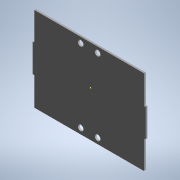
# Autodesk Inventor part: Level1
Saved by Autodesk Inventor 2020 (Build 240168000, 168)
## iProperties
Part Number: Level1
Material: Generic
Document SubType Name: Modeling
Designer: SBBA
Appearance: Default
Mass: 86.85 g
Surface Area: 601.8 cm^2
Volume: 86.85 cm^3
Density: 1 g/cm^3
Author: SBBA
Autodesk Inventor part; units mm, degrees
ref_plane "YZ Plane" through (0, 0, 0) normal (1, 0, 0) x (0, 1, 0)
ref_plane "XZ Plane" through (0, 0, 0) normal (0, 1, 0) x (-1, 0, 0)
ref_plane "XY Plane" through (0, 0, 0) normal (0, 0, 1) x (1, 0, 0)
sketch "Sketch1" plane through (0, 0, 0) normal (0, 0, 1) x (1, 0, 0)
  line L0 (-102.5157, 69.2842) -> (97.4843, 69.2842)
  line L1 (97.4843, 69.2842) -> (97.4843, -80.7158)
  line L2 (97.4843, -80.7158) -> (-102.5157, -80.7158)
  line L3 (-102.5157, -80.7158) -> (-102.5157, 69.2842)
  point P0 (0, 0)
  constraints: 8 end point, 2 parallel, 1 horizontal, 1 perpendicular
extrude "Extrusion1" add sketch "Sketch1" along normal blind 3
sketch "Sketch3" plane through (0, 0, 3) normal (0, 0, 1) x (1, 0, 0)
  point P0 (0, 0)
sketch "Sketch4" plane through (0, 0, 3) normal (0, 0, 1) x (1, 0, 0)
  line L0 (97.4843, 69.2842) -> (-102.5157, 69.2842) projected
  line L1 (-102.5157, 69.2842) -> (-99.5157, 69.2842)
  line L2 (-99.5157, 69.2842) -> (-99.5157, 19.2842)
  line L3 (-99.5157, 19.2842) -> (-102.5157, 19.2842)
  line L4 (-102.5157, 19.2842) -> (-102.5157, 69.2842)
  point P0 (0, 0)
  constraints: 8 end point, 2 parallel, 1 horizontal, 1 perpendicular
extrude "Extrusion2" cut sketch "Sketch4" against normal blind 3
sketch "Sketch5" plane through (0, 0, 3) normal (0, 0, 1) x (1, 0, 0)
  line L0 (97.4843, -80.7158) -> (94.4843, -80.7158)
  line L1 (94.4843, -80.7158) -> (94.4843, -30.7158)
  line L2 (94.4843, -30.7158) -> (97.4843, -30.7158)
  line L3 (97.4843, -30.7158) -> (97.4843, -80.7158)
  point P0 (0, 0)
  point P1 (-102.5157, -80.7158)
  dimension "d17" = 3
  dimension "d18" = 50
  constraints: 8 end point, 2 parallel, 1 horizontal, 1 perpendicular
  measures "d17" distance of L1.end L2.end
  measures "d18" distance of L2.end L0.start
extrude "Extrusion3" cut sketch "Sketch5" against normal blind 3
sketch "Sketch6" plane through (0, 0, 3) normal (0, 0, 1) x (1, 0, 0)
  line L0 (97.4843, -30.7158) -> (97.4843, 69.2842) projected
  line L1 (97.4843, 69.2842) -> (94.4843, 69.2842)
  line L2 (94.4843, 69.2842) -> (94.4843, 19.2842)
  line L3 (94.4843, 19.2842) -> (97.4843, 19.2842)
  line L4 (97.4843, 19.2842) -> (97.4843, 69.2842)
  point P0 (0, 0)
  dimension "d21" = 50
  dimension "d22" = 3
  constraints: 8 end point, 2 parallel, 1 horizontal, 1 perpendicular
  measures "d21" distance of L1.end L2.end
  measures "d22" distance of L0.end L1.end
extrude "Extrusion4" cut sketch "Sketch6" against normal blind 3
sketch "Sketch7" plane through (0, 0, 3) normal (0, 0, 1) x (1, 0, 0)
  line L0 (-102.5157, 19.2842) -> (-102.5157, -80.7158) projected
  line L1 (-102.5157, -80.7158) -> (-99.5157, -80.7158)
  line L2 (-99.5157, -80.7158) -> (-99.5157, -30.7158)
  line L3 (-99.5157, -30.7158) -> (-102.5157, -30.7158)
  line L4 (-102.5157, -30.7158) -> (-102.5157, -80.7158)
  point P0 (0, 0)
  dimension "d25" = 50
  dimension "d26" = 3
  constraints: 8 end point, 2 parallel, 1 horizontal, 1 perpendicular
  measures "d25" distance of L1.end L2.end
  measures "d26" distance of L2.end L3.end
extrude "Extrusion5" cut sketch "Sketch7" against normal blind 3
sketch "Sketch8" plane through (0, 0, 3) normal (0, 0, 1) x (1, 0, 0)
  line L0 (-102.5157, -30.7158) -> (-102.5157, 19.2842) projected
  line L1 (97.4843, -30.7158) -> (94.4843, -30.7158) projected
  line L2 (94.4843, -80.7158) -> (-99.5157, -80.7158) projected
  line L3 (-10.0157, -50.7158) -> (4.9843, -50.7158)
  line L4 (4.9843, -50.7158) -> (4.9843, -80.7158)
  line L5 (4.9843, -80.7158) -> (-10.0157, -80.7158)
  line L6 (-10.0157, -80.7158) -> (-10.0157, -50.7158)
  point P0 (0, 0)
  dimension "d32" = 15
  dimension "d33" = 30
  constraints: 8 end point, 2 parallel, 1 horizontal, 1 perpendicular, 1 point on line
  measures "d32" distance of L3.start L3.end
  measures "d33" distance of L3.end L4.end
extrude "Extrusion6" cut sketch "Sketch8" against normal blind 3
sketch "Sketch9" plane through (-10.0157, -50.7158, 3) normal (0, -1, 0) x (1, 0, 0)
  line L0 (0, 0) -> (15, 0) projected
  line L1 (15, -3) -> (0, -3) projected
  line L2 (0, 0) -> (15, 0)
  line L3 (15, 0) -> (15, -3)
  line L4 (15, -3) -> (0, -3)
  line L5 (0, -3) -> (0, 0)
  point P0 (10.0157, -3)
  constraints: 8 end point, 2 parallel, 1 horizontal, 1 perpendicular
extrude "Extrusion7" add sketch "Sketch9" along normal blind 30
sketch "Sketch10" plane through (0, 0, 0) normal (0, 0, -1) x (-1, 0, 0)
  line L0 (-94.4843, 69.2842) -> (99.5157, 69.2842) projected
  line L1 (99.5157, -80.7158) -> (-94.4843, -80.7158) projected
  line L2 (-97.4843, 19.2842) -> (-97.4843, -30.7158) projected
  line L3 (102.5157, 19.2842) -> (102.5157, -30.7158) projected
  line L4 (2.5157, 69.2842) -> (102.5157, 69.2842)
  circle A0 centre (-12.4843, 59.2842) radius 5
  circle A1 centre (17.5157, 59.2842) radius 5
  circle A2 centre (-12.4843, -70.7158) radius 5
  circle A3 centre (17.5157, -70.7158) radius 5
  point P0 (0, 0)
  constraints: 4 centre point, 2 end point, 1 midpoint, 1 point on line
extrude "Extrusion8" cut sketch "Sketch10" against normal blind 24.75
body "Solid1"
